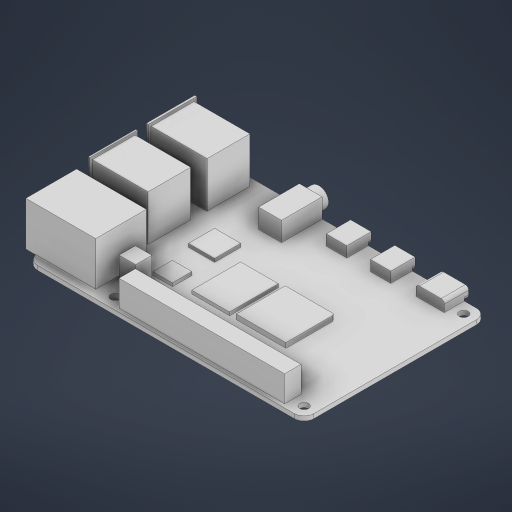
# Autodesk Inventor part: RaspberryPi4
Saved by Autodesk Inventor 2024 (Build 280153000, 153)
## iProperties
Created: 2025-09-25
Part Number: RaspberryPi4
Material: Generic
Document SubType Name: Modeling
Designer: kevin
Density: 1 g/cm^3
Appearance: Default
Author: kevin
Autodesk Inventor part; units mm, degrees
ref_plane "YZ Plane" through (0, 0, 0) normal (1, 0, 0) x (0, 1, 0)
ref_plane "XZ Plane" through (0, 0, 0) normal (0, 1, 0) x (-1, 0, 0)
ref_plane "XY Plane" through (0, 0, 0) normal (0, 0, 1) x (1, 0, 0)
sketch "Sketch2" plane through (0, 0, 0) normal (0, 1, 0) x (-1, 0, 0)
  line L0 (-64.8849, 45.8064) -> (79.608, 45.8064) construction
  line L1 (79.608, 45.8064) -> (79.608, -48.1736) construction
  line L2 (79.608, -48.1736) -> (-64.8849, -48.1736) construction
  line L3 (-64.8849, -48.1736) -> (-64.8849, 45.8064) construction
  point P0 (0, 0)
  dimension "d21" = 93.98
  constraints: 2 other
  measures "d21" distance of L0.end L1.end
sketch "Sketch1" plane through (0, 0, 0) normal (0, 1, 0) x (-1, 0, 0)
  line L0 (-39.5, 28) -> (39.325, 28)
  line L1 (42.5, 24.825) -> (42.5, -25)
  line L2 (39.5, -28) -> (-39.5, -28)
  line L3 (-42.5, -25) -> (-42.5, 25)
  line L4 (-42.5, 28) -> (42.5, -28) construction
  line L5 (42.5, 28) -> (-42.5, -28) construction
  circle A0 centre (-39, 24.5) radius 1.35
  circle A1 centre (-39, 24.5) radius 3
  circle A2 centre (-39, -24.5) radius 3
  circle A3 centre (-39, -24.5) radius 1.35
  circle A4 centre (19, -24.5) radius 1.35
  circle A5 centre (19, -24.5) radius 3
  line L6 (-39, -24.5) -> (20.35, -24.5) construction
  line L7 (19, -24.5) -> (19, 28) construction
  line L8 (19, 24.5) -> (-39, 24.5) construction
  circle A6 centre (19, 24.5) radius 1.35
  circle A7 centre (19, 24.5) radius 3
  arc A8 (42.5, 24.825) -> (39.325, 28) centre (39.325, 24.825) ccw
  arc A9 (39.5, -28) -> (42.5, -25) centre (39.5, -25) ccw
  arc A10 (-42.5, -25) -> (-39.5, -28) centre (-39.5, -25) ccw
  arc A11 (-39.5, 28) -> (-42.5, 25) centre (-39.5, 25) ccw
  point P0 (0, 0)
  dimension "d80" = 2.7
  dimension "d0" = 85
  dimension "d1" = 56
  dimension "d72" = 2.7
  dimension "d73" = 3.5
  dimension "d74" = 3.5
  dimension "d75" = 6
  dimension "d76" = 6
  dimension "d77" = 2.7
  dimension "d78" = 3.5
  dimension "d79" = 3.5
  dimension "d81" = 6
  dimension "d82" = 58
  dimension "d88" = 2.7
  dimension "d89" = 6
  dimension "d90" = 3.175
  dimension "d91" = 3
  constraints: 18 end point, 11 centre point, 11 point on line, 8 point on circle, 8 tangent, 5 coincident, 3 horizontal, 2 equal radius, 2 midpoint, 2 parallel, 2 perpendicular, 1 horizontal alignment, 2 other
  measures "d0" distance of L4.end L5.end
  measures "d1" distance of L5.start L4.end
  measures "d72" diameter of A0
  measures "d73" distance from line of L3 A0.centre
  measures "d74" distance from line of L0 A0.centre
  measures "d75" diameter of A1
  measures "d76" diameter of A2
  measures "d77" diameter of A3
  measures "d78" distance from line of L2 A2.centre
  measures "d79" distance from line of L3 A2.centre
  measures "d81" diameter of A5
  measures "d82" distance of L6.start point (19, -24.5)
  measures "d88" diameter of A6
  measures "d89" diameter of A7
  measures "d90" radius of A8
  measures "d91" radius of A9
extrude "Extrusion1" add sketch "Sketch1" against normal blind 1.35 contours L0 A8 L1 A9 L2 A10 L3 A11 | A1 | A2 | A5 | A7
sketch "Sketch3" plane through (0, 0, 0) normal (0, 1, 0) x (1, 0, 0)
  line L0 (39.5, 28) -> (-39.5, 28) projected
  arc A0 (-39.5, 28) -> (-42.5, 25) centre (-39.5, 25) ccw projected
  line L1 (-42.5, 25) -> (-42.5, -24.825) projected
  arc A1 (-42.5, -24.825) -> (-39.325, -28) centre (-39.325, -24.825) ccw projected
  line L2 (-39.325, -28) -> (39.5, -28) projected
  arc A2 (39.5, -28) -> (42.5, -25) centre (39.5, -25) ccw projected
  line L3 (42.5, -25) -> (42.5, 25) projected
  arc A3 (42.5, 25) -> (39.5, 28) centre (39.5, 25) ccw projected
  circle A4 centre (39, -24.5) radius 1.35 projected
  circle A5 centre (39, 24.5) radius 1.35 projected
  circle A6 centre (-19, 24.5) radius 1.35 projected
  circle A7 centre (-19, -24.5) radius 1.35 projected
  line L4 (-24.0477, -25.4754) -> (-45.4891, -25.4754)
  line L5 (-45.4891, -25.4754) -> (-45.4891, -9.8923)
  line L6 (-45.4891, -9.8923) -> (-24.0477, -9.8923)
  line L7 (-24.0477, -9.8923) -> (-24.0477, -25.4754)
  line L8 (-27.9495, -5.5035) -> (-45.4617, -5.5035)
  line L9 (-45.4617, -5.5035) -> (-45.4617, 7.5977)
  line L10 (-45.4617, 7.5977) -> (-27.9495, 7.5977)
  line L11 (-27.9495, 7.5977) -> (-27.9495, -5.5035)
  line L12 (-27.7191, 12.4037) -> (-45.4891, 12.4037)
  line L13 (-45.4891, 12.4037) -> (-45.4891, 25.5708)
  line L14 (-45.4891, 25.5708) -> (-27.7191, 25.5708)
  line L15 (-27.7191, 25.5708) -> (-27.7191, 12.4037)
  line L16 (35.4341, -26.9217) -> (-15.4304, -26.9217)
  line L17 (-15.4304, -26.9217) -> (-15.4304, -21.8907)
  line L18 (-15.4304, -21.8907) -> (35.4341, -21.8907)
  line L19 (35.4341, -21.8907) -> (35.4341, -26.9217)
  line L20 (-16.4464, -20.7967) -> (-21.5584, -20.7967)
  line L21 (-21.5584, -20.7967) -> (-21.5584, -15.7781)
  line L22 (-21.5584, -15.7781) -> (-16.4464, -15.7781)
  line L23 (-16.4464, -15.7781) -> (-16.4464, -20.7967)
  line L24 (-12.9864, -12.9727) -> (-19.0024, -12.9727)
  line L25 (-19.0024, -12.9727) -> (-19.0024, -6.9567)
  line L26 (-19.0024, -6.9567) -> (-12.9864, -6.9567)
  line L27 (-12.9864, -6.9567) -> (-12.9864, -12.9727)
  line L28 (-12.9864, 0) -> (-21.0285, 0)
  line L29 (-21.0285, 0) -> (-21.0285, 8.0366)
  line L30 (-21.0285, 8.0366) -> (-12.9864, 8.0366)
  line L31 (-12.9864, 8.0366) -> (-12.9864, 0)
  line L32 (3.5343, -11.9441) -> (-8.0925, -11.9441)
  line L33 (-8.0925, -11.9441) -> (-8.0925, 3.0804)
  line L34 (-8.0925, 3.0804) -> (3.5343, 3.0804)
  line L35 (3.5343, 3.0804) -> (3.5343, -11.9441)
  line L36 (20.8342, -11.9441) -> (5.6228, -11.9441)
  line L37 (5.6228, -11.9441) -> (5.6228, 3.0804)
  line L38 (5.6228, 3.0804) -> (20.3355, 3.0804)
  line L39 (20.8342, 2.4881) -> (20.8342, -11.9441)
  line L40 (20.8342, 2.4881) -> (20.3355, 3.0804)
  line L41 (35.6718, 21.889) -> (26.9986, 21.889)
  line L42 (26.9986, 21.889) -> (26.9986, 29.352)
  line L43 (26.9986, 29.352) -> (35.6718, 29.352)
  line L44 (35.6718, 29.352) -> (35.6718, 21.889)
  line L45 (19.6618, 21.4604) -> (13.409, 21.4604)
  line L46 (13.409, 21.4604) -> (13.409, 28.9486)
  line L47 (13.409, 28.9486) -> (19.6618, 28.9486)
  line L48 (19.6618, 28.9486) -> (19.6618, 21.4604)
  line L49 (6.1478, 21.4604) -> (-0.1806, 21.4604)
  line L50 (-0.1806, 21.4604) -> (-0.1806, 28.9486)
  line L51 (-0.1806, 28.9486) -> (6.1478, 28.9486)
  line L52 (6.1478, 28.9486) -> (6.1478, 21.4604)
  line L53 (-7.9514, 15.5003) -> (-14.9702, 15.5003)
  line L54 (-14.9702, 15.5003) -> (-14.9702, 28.1482)
  line L55 (-14.9702, 28.1482) -> (-7.9514, 28.1482)
  line L56 (-7.9514, 28.1482) -> (-7.9514, 15.5003)
  point P0 (0, 0)
  point P1 (-42.5, -9.8923)
  point P2 (-42.4327, -25.4754)
  point P3 (-7.9514, 28)
  point P4 (-14.9702, 28)
  constraints: 106 end point, 26 parallel, 13 horizontal, 13 perpendicular, 5 point on line
extrude "Extrusion2" add sketch "Sketch3" along normal blind 14 contours L8 L9 L10 L1 | L1 L10 L11 L8 | L14 L15 L12 L1 A0 | A0 L1 L12 L13 L14
extrude "Extrusion3" add sketch "Sketch3" along normal blind 13.5 contours L4 L5 L6 L1 A1 | A1 L1 L6 L7 L4
extrude "Extrusion4" add sketch "Sketch3" along normal blind 1.5 contours L36 L37 L38 L40 L39
extrude "Extrusion5" add sketch "Sketch3" along normal blind 1 contours L24 L25 L26 L27 | L28 L29 L30 L31 | L32 L33 L34 L35
extrude "Extrusion6" add sketch "Sketch3" along normal blind 8 contours L16 L17 L18 L19 | L20 L21 L22 L23
extrude "Extrusion7" add sketch "Sketch3" along normal blind 3.22 contours L44 L41 L42 L0 | L0 L42 L43 L44 | L48 L45 L46 L0 | L0 L46 L47 L48 | L52 L49 L50 L0 | L0 L50 L51 L52
extrude "Extrusion8" add sketch "Sketch3" along normal blind 5.922 contours L56 L53 L54 L0
sketch "Sketch4" plane through (39.5, -1.35, -28) normal (0, 0, -1) x (-1, 0, 0)
  line L0 (0, 1.35) -> (3.8282, 1.35) projected
  line L1 (0, 1.35) -> (0, 0) projected
  line L2 (79, 0) -> (0, 0) projected
  line L3 (79, 1.35) -> (79, 0) projected
  line L4 (54.4702, 1.35) -> (79, 1.35) projected
  line L5 (54.4702, 1.35) -> (54.4702, 7.272) projected
  line L6 (47.4514, 7.272) -> (54.4702, 7.272) projected
  line L7 (47.4514, 1.35) -> (47.4514, 7.272) projected
  line L8 (39.6806, 1.35) -> (47.4514, 1.35) projected
  line L9 (33.3522, 1.35) -> (39.6806, 1.35) projected
  line L10 (26.091, 1.35) -> (33.3522, 1.35) projected
  line L11 (19.8382, 1.35) -> (26.091, 1.35) projected
  line L12 (12.5014, 1.35) -> (19.8382, 1.35) projected
  line L13 (3.8282, 1.35) -> (12.5014, 1.35) projected
  line L14 (47.4514, 7.272) -> (54.4702, 1.35) construction
  circle A0 centre (50.9608, 4.311) radius 2.961
  point P0 (39.5, 1.35)
  constraints: 2 end point, 1 centre point, 1 midpoint
extrude "Extrusion9" add sketch "Sketch4" along normal blind 2.5 contours A0
sketch "Sketch5" plane through (0, 0, 0) normal (0, 1, 0) x (1, 0, 0)
  line L0 (-44.9359, 11.6307) -> (-45.5614, 11.6307)
  line L1 (-45.5614, 11.6307) -> (-45.5614, 26.4615)
  line L2 (-45.5614, 26.4615) -> (-44.9359, 26.4615)
  line L3 (-44.9359, 26.4615) -> (-44.9359, 11.6307)
  line L4 (-45.0895, -6.2124) -> (-45.5614, -6.2124)
  line L5 (-45.5614, -6.2124) -> (-45.5614, 8.372)
  line L6 (-45.5614, 8.372) -> (-45.0895, 8.372)
  line L7 (-45.0895, 8.372) -> (-45.0895, -6.2124)
  point P0 (0, 0)
  constraints: 16 end point, 4 parallel, 2 horizontal, 2 perpendicular, 1 point on line
extrude "Extrusion10" add sketch "Sketch5" along normal blind 14.8844 and the other way blind 0.889
sketch "Sketch6" plane through (-45.5614, -0.889, -11.6307) normal (-1, 0, 0) x (0, 0, 1)
  line L0 (0, 0) -> (0, 15.7734) projected
  line L1 (-14.8308, 15.7734) -> (0, 15.7734) projected
  line L2 (-14.8308, 0) -> (-14.8308, 15.7734) projected
  line L3 (0, 0) -> (-14.8308, 0) projected
  line L4 (17.8431, 0) -> (17.8431, 15.7734) projected
  line L5 (3.2587, 15.7734) -> (17.8431, 15.7734) projected
  line L6 (3.2587, 0) -> (3.2587, 15.7734) projected
  line L7 (17.8431, 0) -> (3.2587, 0) projected
  line L8 (-13.3693, 0.889) -> (-0.773, 0.889) projected
  line L9 (-13.3693, 0.889) -> (-13.3693, -0.461) projected
  line L10 (36.4557, -0.461) -> (-13.3693, -0.461) projected
  line L11 (17.1342, 0.889) -> (21.523, 0.889) projected
  line L12 (4.0329, 0.889) -> (17.1342, 0.889) projected
  line L13 (-0.773, 0.889) -> (4.0329, 0.889) projected
  line L14 (-14.8308, 15.7734) -> (0, 0) construction
  line L15 (17.8431, 15.7734) -> (3.2587, 15.7734) construction
  line L16 (3.2587, 15.7734) -> (17.8431, 0) construction
  line L17 (21.523, 14.389) -> (36.4557, 0.889) construction
  line L18 (-13.7436, 1.3844) -> (-1.0873, 1.3844)
  line L19 (-1.0873, 1.3844) -> (-1.0873, 14.389)
  line L20 (-1.0873, 14.389) -> (-13.7436, 14.389)
  line L21 (-13.7436, 14.389) -> (-13.7436, 1.3844)
  line L22 (-13.7436, 1.3844) -> (-1.0873, 14.389) construction
  line L23 (-1.0873, 1.3844) -> (-13.7436, 14.389) construction
  line L24 (4.6502, 1.3844) -> (16.4515, 1.3844)
  line L25 (16.4515, 1.3844) -> (16.4515, 14.389)
  line L26 (16.4515, 14.389) -> (4.6502, 14.389)
  line L27 (4.6502, 14.389) -> (4.6502, 1.3844)
  line L28 (4.6502, 1.3844) -> (16.4515, 14.389) construction
  line L29 (16.4515, 1.3844) -> (4.6502, 14.389) construction
  line L30 (22.6059, 1.4602) -> (35.3727, 1.4602)
  line L31 (35.3727, 1.4602) -> (35.3727, 11.8279)
  line L32 (35.3727, 11.8279) -> (22.6059, 11.8279)
  line L33 (22.6059, 11.8279) -> (22.6059, 1.4602)
  line L34 (22.6059, 1.4602) -> (35.3727, 11.8279) construction
  line L35 (35.3727, 1.4602) -> (22.6059, 11.8279) construction
  line L36 (-13.7436, 6.591) -> (-1.0873, 6.591)
  line L37 (-1.0873, 6.591) -> (-1.0873, 9.1824)
  line L38 (-1.0873, 9.1824) -> (-13.7436, 9.1824)
  line L39 (-13.7436, 9.1824) -> (-13.7436, 6.591)
  line L40 (-13.7436, 6.591) -> (-1.0873, 9.1824) construction
  line L41 (-1.0873, 6.591) -> (-13.7436, 9.1824) construction
  line L42 (4.6502, 6.591) -> (16.4515, 6.591)
  line L43 (16.4515, 6.591) -> (16.4515, 9.1824)
  line L44 (16.4515, 9.1824) -> (4.6502, 9.1824)
  line L45 (4.6502, 9.1824) -> (4.6502, 6.591)
  line L46 (4.6502, 6.591) -> (16.4515, 9.1824) construction
  line L47 (16.4515, 6.591) -> (4.6502, 9.1824) construction
  line L48 (36.4557, 0.889) -> (36.4557, -0.461) projected
  line L49 (21.523, 0.889) -> (36.4557, 0.889) projected
  point P0 (11.6307, 0.889)
  point P1 (-7.4154, 7.8867)
  point P2 (10.5509, 7.8867)
  point P3 (28.9893, 6.644)
  point P4 (-1.0873, 6.591)
  point P5 (-13.7436, 6.591)
  point P6 (-13.7436, 9.1824)
  constraints: 66 end point, 12 midpoint, 10 parallel, 5 horizontal, 5 perpendicular, 4 point on line
extrude "Extrusion11" cut sketch "Sketch6" against normal blind 14.8844 contours L21 L36 L19 L18 | L21 L20 L19 L38 | L27 L42 L25 L24 | L27 L26 L25 L44 | L33 L32 L31 L30
fillet "Fillet1" radius 1 8 edges at (26.9986, 3.22, -25.6205) (35.6718, 3.22, -25.6205) (26.9986, 0, -28.676) (35.6718, 0, -28.676) (19.6618, 0, -28.4743) (13.409, 0, -28.4743) (6.1478, 0, -28.4743) (-0.1806, 0, -28.4743)
equation "\"d80\" = d77"
equation "\"d74\" = d73"
equation "\"d76\" = d75"
equation "\"d77\" = d72"
equation "\"d78\" = d74"
equation "\"d79\" = d78"
equation "\"d81\" = d76"
equation "\"d88\" = d72"
equation "\"d89\" = d75"
body "Solid1"
